Autodesk Fusion 360 part; units mm, degrees
(part 2 of 5)
sketch "Rear engraving master - manufacturing sketch" plane through (0, 0, -4.775) normal (0, 0, 1) x (1, 0, 0) in component "02 Clear acrylic"
  line L0 (17.075, 29.8895) -> (17.0879, 30.5633)
  line L1 (17.0879, 30.5633) -> (17.1264, 31.2094)
  line L2 (17.1264, 31.2094) -> (17.1907, 31.8279)
  line L3 (17.1907, 31.8279) -> (17.2807, 32.4188)
  line L4 (17.2807, 32.4188) -> (17.3964, 32.9821)
  line L5 (17.3964, 32.9821) -> (17.5378, 33.5177)
  line L6 (17.5378, 33.5177) -> (17.7049, 34.0257)
  line L7 (17.7049, 34.0257) -> (17.8977, 34.5061)
  line L8 (17.8977, 34.5061) -> (18.2326, 35.1761)
  line L9 (18.2326, 35.1761) -> (18.6236, 35.8107)
  line L10 (18.6236, 35.8107) -> (19.0706, 36.41)
  line L11 (19.0706, 36.41) -> (19.5737, 36.9741)
  line L12 (19.5737, 36.9741) -> (20.1174, 37.4852)
  line L13 (20.1174, 37.4852) -> (20.6864, 37.9256)
  line L14 (20.6864, 37.9256) -> (21.2807, 38.2955)
  line L15 (21.2807, 38.2955) -> (21.9004, 38.5948)
  line L16 (21.9004, 38.5948) -> (22.329, 38.7617)
  line L17 (22.329, 38.7617) -> (22.7737, 38.9064)
  line L18 (22.7737, 38.9064) -> (23.2345, 39.0288)
  line L19 (23.2345, 39.0288) -> (23.7115, 39.1289)
  line L20 (23.7115, 39.1289) -> (24.2045, 39.2068)
  line L21 (24.2045, 39.2068) -> (24.7137, 39.2624)
  line L22 (24.7137, 39.2624) -> (25.239, 39.2958)
  line L23 (25.239, 39.2958) -> (25.7804, 39.307)
  line L24 (25.7804, 39.307) -> (26.2714, 39.2973)
  line L25 (26.2714, 39.2973) -> (26.7501, 39.2684)
  line L26 (26.7501, 39.2684) -> (27.2163, 39.2202)
  line L27 (27.2163, 39.2202) -> (27.6701, 39.1527)
  line L28 (27.6701, 39.1527) -> (28.1114, 39.0659)
  line L29 (28.1114, 39.0659) -> (28.5404, 38.9599)
  line L30 (28.5404, 38.9599) -> (28.9569, 38.8346)
  line L31 (28.9569, 38.8346) -> (29.361, 38.69)
  line L32 (29.361, 38.69) -> (29.7527, 38.5261)
  line L33 (29.7527, 38.5261) -> (30.132, 38.3429)
  line L34 (30.132, 38.3429) -> (30.4988, 38.1405)
  line L35 (30.4988, 38.1405) -> (30.8532, 37.9187)
  line L36 (30.8532, 37.9187) -> (31.1952, 37.6777)
  line L37 (31.1952, 37.6777) -> (31.5248, 37.4174)
  line L38 (31.5248, 37.4174) -> (31.8419, 37.1379)
  line L39 (31.8419, 37.1379) -> (32.1467, 36.839)
  line L40 (32.1467, 36.839) -> (32.4358, 36.523)
  line L41 (32.4358, 36.523) -> (32.7064, 36.1919)
  line L42 (32.7064, 36.1919) -> (32.9582, 35.8458)
  line L43 (32.9582, 35.8458) -> (33.1915, 35.4846)
  line L44 (33.1915, 35.4846) -> (33.406, 35.1083)
  line L45 (33.406, 35.1083) -> (33.6019, 34.717)
  line L46 (33.6019, 34.717) -> (33.7792, 34.3106)
  line L47 (33.7792, 34.3106) -> (33.9378, 33.8892)
  line L48 (33.9378, 33.8892) -> (34.0777, 33.4526)
  line L49 (34.0777, 33.4526) -> (34.199, 33.0011)
  line L50 (34.199, 33.0011) -> (34.3016, 32.5345)
  line L51 (34.3016, 32.5345) -> (34.3855, 32.0528)
  line L52 (34.3855, 32.0528) -> (34.4508, 31.556)
  line L53 (34.4508, 31.556) -> (34.4975, 31.0442)
  line L54 (34.4975, 31.0442) -> (34.5255, 30.5174)
  line L55 (34.5255, 30.5174) -> (34.5348, 29.9754)
  line L56 (34.5348, 29.9754) -> (34.5255, 29.438)
  line L57 (34.5255, 29.438) -> (34.4978, 28.9154)
  line L58 (34.4978, 28.9154) -> (34.4515, 28.4076)
  line L59 (34.4515, 28.4076) -> (34.3867, 27.9146)
  line L60 (34.3867, 27.9146) -> (34.3034, 27.4364)
  line L61 (34.3034, 27.4364) -> (34.2015, 26.9731)
  line L62 (34.2015, 26.9731) -> (34.0812, 26.5246)
  line L63 (34.0812, 26.5246) -> (33.9424, 26.0909)
  line L64 (33.9424, 26.0909) -> (33.785, 25.672)
  line L65 (33.785, 25.672) -> (33.6091, 25.268)
  line L66 (33.6091, 25.268) -> (33.4147, 24.8787)
  line L67 (33.4147, 24.8787) -> (33.2018, 24.5043)
  line L68 (33.2018, 24.5043) -> (32.9704, 24.1447)
  line L69 (32.9704, 24.1447) -> (32.7205, 23.7999)
  line L70 (32.7205, 23.7999) -> (32.452, 23.47)
  line L71 (32.452, 23.47) -> (32.1651, 23.1548)
  line L72 (32.1651, 23.1548) -> (31.8626, 22.8567)
  line L73 (31.8626, 22.8567) -> (31.5477, 22.5779)
  line L74 (31.5477, 22.5779) -> (31.2203, 22.3182)
  line L75 (31.2203, 22.3182) -> (30.8805, 22.0778)
  line L76 (30.8805, 22.0778) -> (30.5281, 21.8566)
  line L77 (30.5281, 21.8566) -> (30.1633, 21.6547)
  line L78 (30.1633, 21.6547) -> (29.7861, 21.472)
  line L79 (29.7861, 21.472) -> (29.3963, 21.3085)
  line L80 (29.3963, 21.3085) -> (28.9941, 21.1642)
  line L81 (28.9941, 21.1642) -> (28.5794, 21.0392)
  line L82 (28.5794, 21.0392) -> (28.1523, 20.9335)
  line L83 (28.1523, 20.9335) -> (27.7127, 20.8469)
  line L84 (27.7127, 20.8469) -> (27.2606, 20.7796)
  line L85 (27.2606, 20.7796) -> (26.796, 20.7315)
  line L86 (26.796, 20.7315) -> (26.319, 20.7027)
  line L87 (26.319, 20.7027) -> (25.8295, 20.693)
  line L88 (25.8295, 20.693) -> (25.334, 20.7026)
  line L89 (25.334, 20.7026) -> (24.8514, 20.7313)
  line L90 (24.8514, 20.7313) -> (24.3817, 20.7792)
  line L91 (24.3817, 20.7792) -> (23.9248, 20.8461)
  line L92 (23.9248, 20.8461) -> (23.4808, 20.9323)
  line L93 (23.4808, 20.9323) -> (23.0496, 21.0375)
  line L94 (23.0496, 21.0375) -> (22.6313, 21.1619)
  line L95 (22.6313, 21.1619) -> (22.2258, 21.3054)
  line L96 (22.2258, 21.3054) -> (21.8332, 21.4681)
  line L97 (21.8332, 21.4681) -> (21.4534, 21.6499)
  line L98 (21.4534, 21.6499) -> (21.0865, 21.8508)
  line L99 (21.0865, 21.8508) -> (20.7324, 22.0709)
  line L100 (20.7324, 22.0709) -> (20.3912, 22.3101)
  line L101 (20.3912, 22.3101) -> (20.0629, 22.5685)
  line L102 (20.0629, 22.5685) -> (19.7474, 22.8459)
  line L103 (19.7474, 22.8459) -> (19.4447, 23.1426)
  line L104 (19.4447, 23.1426) -> (19.1578, 23.456)
  line L105 (19.1578, 23.456) -> (18.8893, 23.7838)
  line L106 (18.8893, 23.7838) -> (18.6394, 24.1261)
  line L107 (18.6394, 24.1261) -> (18.408, 24.4828)
  line L108 (18.408, 24.4828) -> (18.1951, 24.854)
  line L109 (18.1951, 24.854) -> (18.0007, 25.2396)
  line L110 (18.0007, 25.2396) -> (17.8248, 25.6396)
  line L111 (17.8248, 25.6396) -> (17.6675, 26.0541)
  line L112 (17.6675, 26.0541) -> (17.5286, 26.483)
  line L113 (17.5286, 26.483) -> (17.4083, 26.9263)
  line L114 (17.4083, 26.9263) -> (17.3065, 27.3841)
  line L115 (17.3065, 27.3841) -> (17.2231, 27.8563)
  line L116 (17.2231, 27.8563) -> (17.1583, 28.3429)
  line L117 (17.1583, 28.3429) -> (17.1121, 28.844)
  line L118 (17.1121, 28.844) -> (17.0843, 29.3595)
  line L119 (17.0843, 29.3595) -> (17.075, 29.8895)
  line L120 (20.8199, 30.0123) -> (20.842, 29.2711)
  line L121 (20.842, 29.2711) -> (20.9082, 28.5761)
  line L122 (20.9082, 28.5761) -> (21.0185, 27.9274)
  line L123 (21.0185, 27.9274) -> (21.1729, 27.3249)
  line L124 (21.1729, 27.3249) -> (21.3715, 26.7686)
  line L125 (21.3715, 26.7686) -> (21.6142, 26.2586)
  line L126 (21.6142, 26.2586) -> (21.901, 25.7948)
  line L127 (21.901, 25.7948) -> (22.2319, 25.3772)
  line L128 (22.2319, 25.3772) -> (22.5968, 25.0074)
  line L129 (22.5968, 25.0074) -> (22.9855, 24.6869)
  line L130 (22.9855, 24.6869) -> (23.398, 24.4158)
  line L131 (23.398, 24.4158) -> (23.8342, 24.1939)
  line L132 (23.8342, 24.1939) -> (24.2943, 24.0213)
  line L133 (24.2943, 24.0213) -> (24.7781, 23.8981)
  line L134 (24.7781, 23.8981) -> (25.2858, 23.8241)
  line L135 (25.2858, 23.8241) -> (25.8172, 23.7995)
  line L136 (25.8172, 23.7995) -> (26.3483, 23.8239)
  line L137 (26.3483, 23.8239) -> (26.8551, 23.8973)
  line L138 (26.8551, 23.8973) -> (27.3375, 24.0196)
  line L139 (27.3375, 24.0196) -> (27.7955, 24.1908)
  line L140 (27.7955, 24.1908) -> (28.2292, 24.411)
  line L141 (28.2292, 24.411) -> (28.6385, 24.68)
  line L142 (28.6385, 24.68) -> (29.0235, 24.998)
  line L143 (29.0235, 24.998) -> (29.384, 25.3649)
  line L144 (29.384, 25.3649) -> (29.7107, 25.7808)
  line L145 (29.7107, 25.7808) -> (29.9937, 26.2455)
  line L146 (29.9937, 26.2455) -> (30.2333, 26.7592)
  line L147 (30.2333, 26.7592) -> (30.4292, 27.3218)
  line L148 (30.4292, 27.3218) -> (30.5817, 27.9333)
  line L149 (30.5817, 27.9333) -> (30.6905, 28.5937)
  line L150 (30.6905, 28.5937) -> (30.7558, 29.3031)
  line L151 (30.7558, 29.3031) -> (30.7776, 30.0614)
  line L152 (30.7776, 30.0614) -> (30.7564, 30.8104)
  line L153 (30.7564, 30.8104) -> (30.6928, 31.5102)
  line L154 (30.6928, 31.5102) -> (30.5868, 32.161)
  line L155 (30.5868, 32.161) -> (30.4384, 32.7626)
  line L156 (30.4384, 32.7626) -> (30.2476, 33.3151)
  line L157 (30.2476, 33.3151) -> (30.0145, 33.8186)
  line L158 (30.0145, 33.8186) -> (29.7389, 34.2728)
  line L159 (29.7389, 34.2728) -> (29.4209, 34.678)
  line L160 (29.4209, 34.678) -> (29.0678, 35.0349)
  line L161 (29.0678, 35.0349) -> (28.6869, 35.3441)
  line L162 (28.6869, 35.3441) -> (28.2781, 35.6058)
  line L163 (28.2781, 35.6058) -> (27.8416, 35.8199)
  line L164 (27.8416, 35.8199) -> (27.3772, 35.9864)
  line L165 (27.3772, 35.9864) -> (26.885, 36.1054)
  line L166 (26.885, 36.1054) -> (26.365, 36.1768)
  line L167 (26.365, 36.1768) -> (25.8172, 36.2005)
  line L168 (25.8172, 36.2005) -> (25.2691, 36.1765)
  line L169 (25.2691, 36.1765) -> (24.7482, 36.1042)
  line L170 (24.7482, 36.1042) -> (24.2546, 35.9839)
  line L171 (24.2546, 35.9839) -> (23.7882, 35.8153)
  line L172 (23.7882, 35.8153) -> (23.3491, 35.5986)
  line L173 (23.3491, 35.5986) -> (22.9372, 35.3338)
  line L174 (22.9372, 35.3338) -> (22.5525, 35.0208)
  line L175 (22.5525, 35.0208) -> (22.1951, 34.6596)
  line L176 (22.1951, 34.6596) -> (21.8728, 34.2499)
  line L177 (21.8728, 34.2499) -> (21.5935, 33.7913)
  line L178 (21.5935, 33.7913) -> (21.3571, 33.2838)
  line L179 (21.3571, 33.2838) -> (21.1637, 32.7273)
  line L180 (21.1637, 32.7273) -> (21.0133, 32.1219)
  line L181 (21.0133, 32.1219) -> (20.9059, 31.4676)
  line L182 (20.9059, 31.4676) -> (20.8414, 30.7644)
  line L183 (20.8414, 30.7644) -> (20.8199, 30.0123)
  line L184 (37.4079, 21) -> (37.4079, 39)
  line L185 (37.4079, 39) -> (40.9441, 39)
  line L186 (40.9441, 39) -> (48.311, 26.9795)
  line L187 (48.311, 26.9795) -> (48.311, 39)
  line L188 (48.311, 39) -> (51.6876, 39)
  line L189 (51.6876, 39) -> (51.6876, 21)
  line L190 (51.6876, 21) -> (48.0409, 21)
  line L191 (48.0409, 21) -> (40.7844, 32.7381)
  line L192 (40.7844, 32.7381) -> (40.7844, 21)
  line L193 (40.7844, 21) -> (37.4079, 21)
  line L194 (77.8158, 21) -> (73.8622, 21)
  line L195 (73.8622, 21) -> (72.2906, 25.0887)
  line L196 (72.2906, 25.0887) -> (65.0955, 25.0887)
  line L197 (65.0955, 25.0887) -> (63.6098, 21)
  line L198 (63.6098, 21) -> (59.7544, 21)
  line L199 (59.7544, 21) -> (66.7653, 39)
  line L200 (66.7653, 39) -> (70.6085, 39)
  line L201 (70.6085, 39) -> (77.8158, 21)
  line L202 (71.1241, 28.1214) -> (68.6439, 34.8008)
  line L203 (68.6439, 34.8008) -> (66.2128, 28.1214)
  line L204 (66.2128, 28.1214) -> (71.1241, 28.1214)
  line L205 (79.633, 21) -> (79.633, 39)
  line L206 (79.633, 39) -> (83.2674, 39)
  line L207 (83.2674, 39) -> (83.2674, 21)
  line L208 (83.2674, 21) -> (79.633, 21)
  line L209 (86.7422, 21) -> (86.7422, 39)
  line L210 (86.7422, 39) -> (94.3915, 39)
  line L211 (94.3915, 39) -> (95.0882, 38.9924)
  line L212 (95.0882, 38.9924) -> (95.7356, 38.9697)
  line L213 (95.7356, 38.9697) -> (96.3337, 38.9318)
  line L214 (96.3337, 38.9318) -> (96.8825, 38.8787)
  line L215 (96.8825, 38.8787) -> (97.382, 38.8105)
  line L216 (97.382, 38.8105) -> (97.8321, 38.7272)
  line L217 (97.8321, 38.7272) -> (98.233, 38.6287)
  line L218 (98.233, 38.6287) -> (98.5846, 38.515)
  line L219 (98.5846, 38.515) -> (98.9033, 38.382)
  line L220 (98.9033, 38.382) -> (99.2058, 38.2253)
  line L221 (99.2058, 38.2253) -> (99.4919, 38.0451)
  line L222 (99.4919, 38.0451) -> (99.7618, 37.8412)
  line L223 (99.7618, 37.8412) -> (100.0153, 37.6138)
  line L224 (100.0153, 37.6138) -> (100.2525, 37.3628)
  line L225 (100.2525, 37.3628) -> (100.4734, 37.0881)
  line L226 (100.4734, 37.0881) -> (100.678, 36.7899)
  line L227 (100.678, 36.7899) -> (100.8622, 36.4743)
  line L228 (100.8622, 36.4743) -> (101.0218, 36.1476)
  line L229 (101.0218, 36.1476) -> (101.1569, 35.8097)
  line L230 (101.1569, 35.8097) -> (101.2674, 35.4608)
  line L231 (101.2674, 35.4608) -> (101.3533, 35.1007)
  line L232 (101.3533, 35.1007) -> (101.4147, 34.7294)
  line L233 (101.4147, 34.7294) -> (101.4516, 34.3471)
  line L234 (101.4516, 34.3471) -> (101.4638, 33.9536)
  line L235 (101.4638, 33.9536) -> (101.4452, 33.4582)
  line L236 (101.4452, 33.4582) -> (101.3894, 32.9848)
  line L237 (101.3894, 32.9848) -> (101.2964, 32.5335)
  line L238 (101.2964, 32.5335) -> (101.1661, 32.1042)
  line L239 (101.1661, 32.1042) -> (100.9986, 31.697)
  line L240 (100.9986, 31.697) -> (100.7939, 31.3119)
  line L241 (100.7939, 31.3119) -> (100.552, 30.9488)
  line L242 (100.552, 30.9488) -> (100.2728, 30.6078)
  line L243 (100.2728, 30.6078) -> (99.9567, 30.293)
  line L244 (99.9567, 30.293) -> (99.6037, 30.0088)
  line L245 (99.6037, 30.0088) -> (99.2138, 29.7551)
  line L246 (99.2138, 29.7551) -> (98.7872, 29.5319)
  line L247 (98.7872, 29.5319) -> (98.3237, 29.3392)
  line L248 (98.3237, 29.3392) -> (97.8233, 29.177)
  line L249 (97.8233, 29.177) -> (97.2861, 29.0453)
  line L250 (97.2861, 29.0453) -> (96.7121, 28.9441)
  line L251 (96.7121, 28.9441) -> (97.2758, 28.5918)
  line L252 (97.2758, 28.5918) -> (97.788, 28.2227)
  line L253 (97.788, 28.2227) -> (98.2488, 27.8367)
  line L254 (98.2488, 27.8367) -> (98.6582, 27.4338)
  line L255 (98.6582, 27.4338) -> (98.8584, 27.2082)
  line L256 (98.8584, 27.2082) -> (99.0753, 26.9427)
  line L257 (99.0753, 26.9427) -> (99.3089, 26.6373)
  line L258 (99.3089, 26.6373) -> (99.5592, 26.2919)
  line L259 (99.5592, 26.2919) -> (99.8261, 25.9067)
  line L260 (99.8261, 25.9067) -> (100.1098, 25.4816)
  line L261 (100.1098, 25.4816) -> (100.4101, 25.0165)
  line L262 (100.4101, 25.0165) -> (100.7271, 24.5116)
  line L263 (100.7271, 24.5116) -> (102.925, 21)
  line L264 (102.925, 21) -> (98.5784, 21)
  line L265 (98.5784, 21) -> (95.9509, 24.9168)
  line L266 (95.9509, 24.9168) -> (95.6148, 25.4174)
  line L267 (95.6148, 25.4174) -> (95.3063, 25.8695)
  line L268 (95.3063, 25.8695) -> (95.0254, 26.2731)
  line L269 (95.0254, 26.2731) -> (94.7722, 26.6281)
  line L270 (94.7722, 26.6281) -> (94.5465, 26.9345)
  line L271 (94.5465, 26.9345) -> (94.3486, 27.1925)
  line L272 (94.3486, 27.1925) -> (94.1782, 27.4019)
  line L273 (94.1782, 27.4019) -> (94.0355, 27.5628)
  line L274 (94.0355, 27.5628) -> (93.7738, 27.8145)
  line L275 (93.7738, 27.8145) -> (93.5044, 28.0232)
  line L276 (93.5044, 28.0232) -> (93.2274, 28.1889)
  line L277 (93.2274, 28.1889) -> (92.9427, 28.3117)
  line L278 (92.9427, 28.3117) -> (92.7879, 28.3592)
  line L279 (92.7879, 28.3592) -> (92.612, 28.4004)
  line L280 (92.612, 28.4004) -> (92.4149, 28.4352)
  line L281 (92.4149, 28.4352) -> (92.1968, 28.4637)
  line L282 (92.1968, 28.4637) -> (91.9576, 28.4858)
  line L283 (91.9576, 28.4858) -> (91.6972, 28.5017)
  line L284 (91.6972, 28.5017) -> (91.4158, 28.5112)
  line L285 (91.4158, 28.5112) -> (91.1132, 28.5143)
  line L286 (91.1132, 28.5143) -> (90.3765, 28.5143)
  line L287 (90.3765, 28.5143) -> (90.3765, 21)
  line L288 (90.3765, 21) -> (86.7422, 21)
  line L289 (90.3765, 31.3874) -> (93.0655, 31.3874)
  line L290 (93.0655, 31.3874) -> (93.6886, 31.3909)
  line L291 (93.6886, 31.3909) -> (94.2503, 31.4013)
  line L292 (94.2503, 31.4013) -> (94.7507, 31.4185)
  line L293 (94.7507, 31.4185) -> (95.1896, 31.4427)
  line L294 (95.1896, 31.4427) -> (95.5672, 31.4738)
  line L295 (95.5672, 31.4738) -> (95.8834, 31.5118)
  line L296 (95.8834, 31.5118) -> (96.1381, 31.5567)
  line L297 (96.1381, 31.5567) -> (96.3315, 31.6085)
  line L298 (96.3315, 31.6085) -> (96.6392, 31.7389)
  line L299 (96.6392, 31.7389) -> (96.9117, 31.9093)
  line L300 (96.9117, 31.9093) -> (97.1488, 32.1195)
  line L301 (97.1488, 32.1195) -> (97.3506, 32.3697)
  line L302 (97.3506, 32.3697) -> (97.5118, 32.6567)
  line L303 (97.5118, 32.6567) -> (97.6269, 32.9775)
  line L304 (97.6269, 32.9775) -> (97.6959, 33.332)
  line L305 (97.6959, 33.332) -> (97.719, 33.7203)
  line L306 (97.719, 33.7203) -> (97.6886, 34.1528)
  line L307 (97.6886, 34.1528) -> (97.5977, 34.5414)
  line L308 (97.5977, 34.5414) -> (97.4461, 34.8864)
  line L309 (97.4461, 34.8864) -> (97.234, 35.1876)
  line L310 (97.234, 35.1876) -> (96.9665, 35.4412)
  line L311 (96.9665, 35.4412) -> (96.6492, 35.6434)
  line L312 (96.6492, 35.6434) -> (96.282, 35.7942)
  line L313 (96.282, 35.7942) -> (95.8649, 35.8936)
  line L314 (95.8649, 35.8936) -> (95.7268, 35.908)
  line L315 (95.7268, 35.908) -> (95.5334, 35.9204)
  line L316 (95.5334, 35.9204) -> (95.2848, 35.931)
  line L317 (95.2848, 35.931) -> (94.9809, 35.9396)
  line L318 (94.9809, 35.9396) -> (94.6218, 35.9463)
  line L319 (94.6218, 35.9463) -> (94.2074, 35.9511)
  line L320 (94.2074, 35.9511) -> (93.7377, 35.954)
  line L321 (93.7377, 35.954) -> (93.2128, 35.955)
  line L322 (93.2128, 35.955) -> (90.3765, 35.955)
  line L323 (90.3765, 35.955) -> (90.3765, 31.3874)
ref_plane "WorkPlane1" through (0, 0, -5.675) normal (0, 0, 1) x (1, 0, 0) in component "03 Registered graphic backing"
sketch "Keyed graphic outline" plane through (0, 0, -5.675) normal (0, 0, 1) x (1, 0, 0) in component "03 Registered graphic backing"
  line L0 (8, 11) -> (112, 11)
  line L1 (112, 11) -> (112, 49)
  line L2 (112, 49) -> (11, 49)
  line L3 (11, 49) -> (8, 46)
  line L4 (8, 46) -> (8, 11)
extrude "Black substrate" add sketch "Keyed graphic outline" against normal blind 1.6 separate body makes body 35 in component "03 Registered graphic backing"
ref_plane "WorkPlane2" through (0, 0, -5.675) normal (0, 0, 1) x (1, 0, 0) in component "03 Registered graphic backing"
sketch "Letter outer 0" plane through (0, 0, -5.675) normal (0, 0, 1) x (1, 0, 0) in component "03 Registered graphic backing"
  line L0 (17.075, 29.8895) -> (17.0879, 30.5633)
  line L1 (17.0879, 30.5633) -> (17.1264, 31.2094)
  line L2 (17.1264, 31.2094) -> (17.1907, 31.8279)
  line L3 (17.1907, 31.8279) -> (17.2807, 32.4188)
  line L4 (17.2807, 32.4188) -> (17.3964, 32.9821)
  line L5 (17.3964, 32.9821) -> (17.5378, 33.5177)
  line L6 (17.5378, 33.5177) -> (17.7049, 34.0257)
  line L7 (17.7049, 34.0257) -> (17.8977, 34.5061)
  line L8 (17.8977, 34.5061) -> (18.2326, 35.1761)
  line L9 (18.2326, 35.1761) -> (18.6236, 35.8107)
  line L10 (18.6236, 35.8107) -> (19.0706, 36.41)
  line L11 (19.0706, 36.41) -> (19.5737, 36.9741)
  line L12 (19.5737, 36.9741) -> (20.1174, 37.4852)
  line L13 (20.1174, 37.4852) -> (20.6864, 37.9256)
  line L14 (20.6864, 37.9256) -> (21.2807, 38.2955)
  line L15 (21.2807, 38.2955) -> (21.9004, 38.5948)
  line L16 (21.9004, 38.5948) -> (22.329, 38.7617)
  line L17 (22.329, 38.7617) -> (22.7737, 38.9064)
  line L18 (22.7737, 38.9064) -> (23.2345, 39.0288)
  line L19 (23.2345, 39.0288) -> (23.7115, 39.1289)
  line L20 (23.7115, 39.1289) -> (24.2045, 39.2068)
  line L21 (24.2045, 39.2068) -> (24.7137, 39.2624)
  line L22 (24.7137, 39.2624) -> (25.239, 39.2958)
  line L23 (25.239, 39.2958) -> (25.7804, 39.307)
  line L24 (25.7804, 39.307) -> (26.2714, 39.2973)
  line L25 (26.2714, 39.2973) -> (26.7501, 39.2684)
  line L26 (26.7501, 39.2684) -> (27.2163, 39.2202)
  line L27 (27.2163, 39.2202) -> (27.6701, 39.1527)
  line L28 (27.6701, 39.1527) -> (28.1114, 39.0659)
  line L29 (28.1114, 39.0659) -> (28.5404, 38.9599)
  line L30 (28.5404, 38.9599) -> (28.9569, 38.8346)
  line L31 (28.9569, 38.8346) -> (29.361, 38.69)
  line L32 (29.361, 38.69) -> (29.7527, 38.5261)
  line L33 (29.7527, 38.5261) -> (30.132, 38.3429)
  line L34 (30.132, 38.3429) -> (30.4988, 38.1405)
  line L35 (30.4988, 38.1405) -> (30.8532, 37.9187)
  line L36 (30.8532, 37.9187) -> (31.1952, 37.6777)
  line L37 (31.1952, 37.6777) -> (31.5248, 37.4174)
  line L38 (31.5248, 37.4174) -> (31.8419, 37.1379)
  line L39 (31.8419, 37.1379) -> (32.1467, 36.839)
  line L40 (32.1467, 36.839) -> (32.4358, 36.523)
  line L41 (32.4358, 36.523) -> (32.7064, 36.1919)
  line L42 (32.7064, 36.1919) -> (32.9582, 35.8458)
  line L43 (32.9582, 35.8458) -> (33.1915, 35.4846)
  line L44 (33.1915, 35.4846) -> (33.406, 35.1083)
  line L45 (33.406, 35.1083) -> (33.6019, 34.717)
  line L46 (33.6019, 34.717) -> (33.7792, 34.3106)
  line L47 (33.7792, 34.3106) -> (33.9378, 33.8892)
  line L48 (33.9378, 33.8892) -> (34.0777, 33.4526)
  line L49 (34.0777, 33.4526) -> (34.199, 33.0011)
  line L50 (34.199, 33.0011) -> (34.3016, 32.5345)
  line L51 (34.3016, 32.5345) -> (34.3855, 32.0528)
  line L52 (34.3855, 32.0528) -> (34.4508, 31.556)
  line L53 (34.4508, 31.556) -> (34.4975, 31.0442)
  line L54 (34.4975, 31.0442) -> (34.5255, 30.5174)
  line L55 (34.5255, 30.5174) -> (34.5348, 29.9754)
  line L56 (34.5348, 29.9754) -> (34.5255, 29.438)
  line L57 (34.5255, 29.438) -> (34.4978, 28.9154)
  line L58 (34.4978, 28.9154) -> (34.4515, 28.4076)
  line L59 (34.4515, 28.4076) -> (34.3867, 27.9146)
  line L60 (34.3867, 27.9146) -> (34.3034, 27.4364)
  line L61 (34.3034, 27.4364) -> (34.2015, 26.9731)
  line L62 (34.2015, 26.9731) -> (34.0812, 26.5246)
  line L63 (34.0812, 26.5246) -> (33.9424, 26.0909)
  line L64 (33.9424, 26.0909) -> (33.785, 25.672)
  line L65 (33.785, 25.672) -> (33.6091, 25.268)
  line L66 (33.6091, 25.268) -> (33.4147, 24.8787)
  line L67 (33.4147, 24.8787) -> (33.2018, 24.5043)
  line L68 (33.2018, 24.5043) -> (32.9704, 24.1447)
  line L69 (32.9704, 24.1447) -> (32.7205, 23.7999)
  line L70 (32.7205, 23.7999) -> (32.452, 23.47)
  line L71 (32.452, 23.47) -> (32.1651, 23.1548)
  line L72 (32.1651, 23.1548) -> (31.8626, 22.8567)
  line L73 (31.8626, 22.8567) -> (31.5477, 22.5779)
  line L74 (31.5477, 22.5779) -> (31.2203, 22.3182)
  line L75 (31.2203, 22.3182) -> (30.8805, 22.0778)
  line L76 (30.8805, 22.0778) -> (30.5281, 21.8566)
  line L77 (30.5281, 21.8566) -> (30.1633, 21.6547)
  line L78 (30.1633, 21.6547) -> (29.7861, 21.472)
  line L79 (29.7861, 21.472) -> (29.3963, 21.3085)
  line L80 (29.3963, 21.3085) -> (28.9941, 21.1642)
  line L81 (28.9941, 21.1642) -> (28.5794, 21.0392)
  line L82 (28.5794, 21.0392) -> (28.1523, 20.9335)
  line L83 (28.1523, 20.9335) -> (27.7127, 20.8469)
  line L84 (27.7127, 20.8469) -> (27.2606, 20.7796)
  line L85 (27.2606, 20.7796) -> (26.796, 20.7315)
  line L86 (26.796, 20.7315) -> (26.319, 20.7027)
  line L87 (26.319, 20.7027) -> (25.8295, 20.693)
  line L88 (25.8295, 20.693) -> (25.334, 20.7026)
  line L89 (25.334, 20.7026) -> (24.8514, 20.7313)
  line L90 (24.8514, 20.7313) -> (24.3817, 20.7792)
  line L91 (24.3817, 20.7792) -> (23.9248, 20.8461)
  line L92 (23.9248, 20.8461) -> (23.4808, 20.9323)
  line L93 (23.4808, 20.9323) -> (23.0496, 21.0375)
  line L94 (23.0496, 21.0375) -> (22.6313, 21.1619)
  line L95 (22.6313, 21.1619) -> (22.2258, 21.3054)
  line L96 (22.2258, 21.3054) -> (21.8332, 21.4681)
  line L97 (21.8332, 21.4681) -> (21.4534, 21.6499)
  line L98 (21.4534, 21.6499) -> (21.0865, 21.8508)
  line L99 (21.0865, 21.8508) -> (20.7324, 22.0709)
  line L100 (20.7324, 22.0709) -> (20.3912, 22.3101)
  line L101 (20.3912, 22.3101) -> (20.0629, 22.5685)
  line L102 (20.0629, 22.5685) -> (19.7474, 22.8459)
  line L103 (19.7474, 22.8459) -> (19.4447, 23.1426)
  line L104 (19.4447, 23.1426) -> (19.1578, 23.456)
  line L105 (19.1578, 23.456) -> (18.8893, 23.7838)
  line L106 (18.8893, 23.7838) -> (18.6394, 24.1261)
  line L107 (18.6394, 24.1261) -> (18.408, 24.4828)
  line L108 (18.408, 24.4828) -> (18.1951, 24.854)
  line L109 (18.1951, 24.854) -> (18.0007, 25.2396)
  line L110 (18.0007, 25.2396) -> (17.8248, 25.6396)
  line L111 (17.8248, 25.6396) -> (17.6675, 26.0541)
  line L112 (17.6675, 26.0541) -> (17.5286, 26.483)
  line L113 (17.5286, 26.483) -> (17.4083, 26.9263)
  line L114 (17.4083, 26.9263) -> (17.3065, 27.3841)
  line L115 (17.3065, 27.3841) -> (17.2231, 27.8563)
  line L116 (17.2231, 27.8563) -> (17.1583, 28.3429)
  line L117 (17.1583, 28.3429) -> (17.1121, 28.844)
  line L118 (17.1121, 28.844) -> (17.0843, 29.3595)
  line L119 (17.0843, 29.3595) -> (17.075, 29.8895)
extrude "Raised letter 0" add sketch "Letter outer 0" along normal blind 0.4 separate body makes body 36 in component "03 Registered graphic backing"
ref_plane "WorkPlane3" through (0, 0, -5.675) normal (0, 0, 1) x (1, 0, 0) in component "03 Registered graphic backing"
sketch "Letter outer 2" plane through (0, 0, -5.675) normal (0, 0, 1) x (1, 0, 0) in component "03 Registered graphic backing"
  line L0 (37.4079, 21) -> (37.4079, 39)
  line L1 (37.4079, 39) -> (40.9441, 39)
  line L2 (40.9441, 39) -> (48.311, 26.9795)
  line L3 (48.311, 26.9795) -> (48.311, 39)
  line L4 (48.311, 39) -> (51.6876, 39)
  line L5 (51.6876, 39) -> (51.6876, 21)
  line L6 (51.6876, 21) -> (48.0409, 21)
  line L7 (48.0409, 21) -> (40.7844, 32.7381)
  line L8 (40.7844, 32.7381) -> (40.7844, 21)
  line L9 (40.7844, 21) -> (37.4079, 21)
extrude "Raised letter 2" add sketch "Letter outer 2" along normal blind 0.4 separate body makes body 37 in component "03 Registered graphic backing"
ref_plane "WorkPlane4" through (0, 0, -5.675) normal (0, 0, 1) x (1, 0, 0) in component "03 Registered graphic backing"
sketch "Letter outer 3" plane through (0, 0, -5.675) normal (0, 0, 1) x (1, 0, 0) in component "03 Registered graphic backing"
  line L0 (77.8158, 21) -> (73.8622, 21)
  line L1 (73.8622, 21) -> (72.2906, 25.0887)
  line L2 (72.2906, 25.0887) -> (65.0955, 25.0887)
  line L3 (65.0955, 25.0887) -> (63.6098, 21)
  line L4 (63.6098, 21) -> (59.7544, 21)
  line L5 (59.7544, 21) -> (66.7653, 39)
  line L6 (66.7653, 39) -> (70.6085, 39)
  line L7 (70.6085, 39) -> (77.8158, 21)
extrude "Raised letter 3" add sketch "Letter outer 3" along normal blind 0.4 separate body makes body 38 in component "03 Registered graphic backing"
ref_plane "WorkPlane5" through (0, 0, -5.675) normal (0, 0, 1) x (1, 0, 0) in component "03 Registered graphic backing"
sketch "Letter outer 5" plane through (0, 0, -5.675) normal (0, 0, 1) x (1, 0, 0) in component "03 Registered graphic backing"
  line L0 (79.633, 21) -> (79.633, 39)
  line L1 (79.633, 39) -> (83.2674, 39)
  line L2 (83.2674, 39) -> (83.2674, 21)
  line L3 (83.2674, 21) -> (79.633, 21)
extrude "Raised letter 5" add sketch "Letter outer 5" along normal blind 0.4 separate body makes body 39 in component "03 Registered graphic backing"
ref_plane "WorkPlane6" through (0, 0, -5.675) normal (0, 0, 1) x (1, 0, 0) in component "03 Registered graphic backing"
sketch "Letter outer 6" plane through (0, 0, -5.675) normal (0, 0, 1) x (1, 0, 0) in component "03 Registered graphic backing"
  line L0 (86.7422, 21) -> (86.7422, 39)
  line L1 (86.7422, 39) -> (94.3915, 39)
  line L2 (94.3915, 39) -> (95.0882, 38.9924)
  line L3 (95.0882, 38.9924) -> (95.7356, 38.9697)
  line L4 (95.7356, 38.9697) -> (96.3337, 38.9318)
  line L5 (96.3337, 38.9318) -> (96.8825, 38.8787)
  line L6 (96.8825, 38.8787) -> (97.382, 38.8105)
  line L7 (97.382, 38.8105) -> (97.8321, 38.7272)
  line L8 (97.8321, 38.7272) -> (98.233, 38.6287)
  line L9 (98.233, 38.6287) -> (98.5846, 38.515)
  line L10 (98.5846, 38.515) -> (98.9033, 38.382)
  line L11 (98.9033, 38.382) -> (99.2058, 38.2253)
  line L12 (99.2058, 38.2253) -> (99.4919, 38.0451)
  line L13 (99.4919, 38.0451) -> (99.7618, 37.8412)
  line L14 (99.7618, 37.8412) -> (100.0153, 37.6138)
  line L15 (100.0153, 37.6138) -> (100.2525, 37.3628)
  line L16 (100.2525, 37.3628) -> (100.4734, 37.0881)
  line L17 (100.4734, 37.0881) -> (100.678, 36.7899)
  line L18 (100.678, 36.7899) -> (100.8622, 36.4743)
  line L19 (100.8622, 36.4743) -> (101.0218, 36.1476)
  line L20 (101.0218, 36.1476) -> (101.1569, 35.8097)
  line L21 (101.1569, 35.8097) -> (101.2674, 35.4608)
  line L22 (101.2674, 35.4608) -> (101.3533, 35.1007)
  line L23 (101.3533, 35.1007) -> (101.4147, 34.7294)
  line L24 (101.4147, 34.7294) -> (101.4516, 34.3471)
  line L25 (101.4516, 34.3471) -> (101.4638, 33.9536)
  line L26 (101.4638, 33.9536) -> (101.4452, 33.4582)
  line L27 (101.4452, 33.4582) -> (101.3894, 32.9848)
  line L28 (101.3894, 32.9848) -> (101.2964, 32.5335)
  line L29 (101.2964, 32.5335) -> (101.1661, 32.1042)
  line L30 (101.1661, 32.1042) -> (100.9986, 31.697)
  line L31 (100.9986, 31.697) -> (100.7939, 31.3119)
  line L32 (100.7939, 31.3119) -> (100.552, 30.9488)
  line L33 (100.552, 30.9488) -> (100.2728, 30.6078)
  line L34 (100.2728, 30.6078) -> (99.9567, 30.293)
  line L35 (99.9567, 30.293) -> (99.6037, 30.0088)
  line L36 (99.6037, 30.0088) -> (99.2138, 29.7551)
  line L37 (99.2138, 29.7551) -> (98.7872, 29.5319)
  line L38 (98.7872, 29.5319) -> (98.3237, 29.3392)
  line L39 (98.3237, 29.3392) -> (97.8233, 29.177)
  line L40 (97.8233, 29.177) -> (97.2861, 29.0453)
  line L41 (97.2861, 29.0453) -> (96.7121, 28.9441)
  line L42 (96.7121, 28.9441) -> (97.2758, 28.5918)
  line L43 (97.2758, 28.5918) -> (97.788, 28.2227)
  line L44 (97.788, 28.2227) -> (98.2488, 27.8367)
  line L45 (98.2488, 27.8367) -> (98.6582, 27.4338)
  line L46 (98.6582, 27.4338) -> (98.8584, 27.2082)
  line L47 (98.8584, 27.2082) -> (99.0753, 26.9427)
  line L48 (99.0753, 26.9427) -> (99.3089, 26.6373)
  line L49 (99.3089, 26.6373) -> (99.5592, 26.2919)
  line L50 (99.5592, 26.2919) -> (99.8261, 25.9067)
  line L51 (99.8261, 25.9067) -> (100.1098, 25.4816)
  line L52 (100.1098, 25.4816) -> (100.4101, 25.0165)
  line L53 (100.4101, 25.0165) -> (100.7271, 24.5116)
  line L54 (100.7271, 24.5116) -> (102.925, 21)
  line L55 (102.925, 21) -> (98.5784, 21)
  line L56 (98.5784, 21) -> (95.9509, 24.9168)
  line L57 (95.9509, 24.9168) -> (95.6148, 25.4174)
  line L58 (95.6148, 25.4174) -> (95.3063, 25.8695)
  line L59 (95.3063, 25.8695) -> (95.0254, 26.2731)
  line L60 (95.0254, 26.2731) -> (94.7722, 26.6281)
  line L61 (94.7722, 26.6281) -> (94.5465, 26.9345)
  line L62 (94.5465, 26.9345) -> (94.3486, 27.1925)
  line L63 (94.3486, 27.1925) -> (94.1782, 27.4019)
  line L64 (94.1782, 27.4019) -> (94.0355, 27.5628)
  line L65 (94.0355, 27.5628) -> (93.7738, 27.8145)
  line L66 (93.7738, 27.8145) -> (93.5044, 28.0232)
  line L67 (93.5044, 28.0232) -> (93.2274, 28.1889)
  line L68 (93.2274, 28.1889) -> (92.9427, 28.3117)
  line L69 (92.9427, 28.3117) -> (92.7879, 28.3592)
  line L70 (92.7879, 28.3592) -> (92.612, 28.4004)
  line L71 (92.612, 28.4004) -> (92.4149, 28.4352)
  line L72 (92.4149, 28.4352) -> (92.1968, 28.4637)
  line L73 (92.1968, 28.4637) -> (91.9576, 28.4858)
  line L74 (91.9576, 28.4858) -> (91.6972, 28.5017)
  line L75 (91.6972, 28.5017) -> (91.4158, 28.5112)
  line L76 (91.4158, 28.5112) -> (91.1132, 28.5143)
  line L77 (91.1132, 28.5143) -> (90.3765, 28.5143)
  line L78 (90.3765, 28.5143) -> (90.3765, 21)
  line L79 (90.3765, 21) -> (86.7422, 21)
extrude "Raised letter 6" add sketch "Letter outer 6" along normal blind 0.4 separate body makes body 40 in component "03 Registered graphic backing"
combine "Union manufactured solid'" operation add target body 35 tool bodies 36 37 38 39 40 in component "03 Registered graphic backing"
ref_plane "WorkPlane7" through (0, 0, -5.275) normal (0, 0, 1) x (1, 0, 0) in component "03 Registered graphic backing"
sketch "Letter counter 1" plane through (0, 0, -5.275) normal (0, 0, 1) x (1, 0, 0) in component "03 Registered graphic backing"
  line L0 (20.8199, 30.0123) -> (20.842, 29.2711)
  line L1 (20.842, 29.2711) -> (20.9082, 28.5761)
  line L2 (20.9082, 28.5761) -> (21.0185, 27.9274)
  line L3 (21.0185, 27.9274) -> (21.1729, 27.3249)
  line L4 (21.1729, 27.3249) -> (21.3715, 26.7686)
  line L5 (21.3715, 26.7686) -> (21.6142, 26.2586)
  line L6 (21.6142, 26.2586) -> (21.901, 25.7948)
  line L7 (21.901, 25.7948) -> (22.2319, 25.3772)
  line L8 (22.2319, 25.3772) -> (22.5968, 25.0074)
  line L9 (22.5968, 25.0074) -> (22.9855, 24.6869)
  line L10 (22.9855, 24.6869) -> (23.398, 24.4158)
  line L11 (23.398, 24.4158) -> (23.8342, 24.1939)
  line L12 (23.8342, 24.1939) -> (24.2943, 24.0213)
  line L13 (24.2943, 24.0213) -> (24.7781, 23.8981)
  line L14 (24.7781, 23.8981) -> (25.2858, 23.8241)
  line L15 (25.2858, 23.8241) -> (25.8172, 23.7995)
  line L16 (25.8172, 23.7995) -> (26.3483, 23.8239)
  line L17 (26.3483, 23.8239) -> (26.8551, 23.8973)
  line L18 (26.8551, 23.8973) -> (27.3375, 24.0196)
  line L19 (27.3375, 24.0196) -> (27.7955, 24.1908)
  line L20 (27.7955, 24.1908) -> (28.2292, 24.411)
  line L21 (28.2292, 24.411) -> (28.6385, 24.68)
  line L22 (28.6385, 24.68) -> (29.0235, 24.998)
  line L23 (29.0235, 24.998) -> (29.384, 25.3649)
  line L24 (29.384, 25.3649) -> (29.7107, 25.7808)
  line L25 (29.7107, 25.7808) -> (29.9937, 26.2455)
  line L26 (29.9937, 26.2455) -> (30.2333, 26.7592)
  line L27 (30.2333, 26.7592) -> (30.4292, 27.3218)
  line L28 (30.4292, 27.3218) -> (30.5817, 27.9333)
  line L29 (30.5817, 27.9333) -> (30.6905, 28.5937)
  line L30 (30.6905, 28.5937) -> (30.7558, 29.3031)
  line L31 (30.7558, 29.3031) -> (30.7776, 30.0614)
  line L32 (30.7776, 30.0614) -> (30.7564, 30.8104)
  line L33 (30.7564, 30.8104) -> (30.6928, 31.5102)
  line L34 (30.6928, 31.5102) -> (30.5868, 32.161)
  line L35 (30.5868, 32.161) -> (30.4384, 32.7626)
  line L36 (30.4384, 32.7626) -> (30.2476, 33.3151)
  line L37 (30.2476, 33.3151) -> (30.0145, 33.8186)
  line L38 (30.0145, 33.8186) -> (29.7389, 34.2728)
  line L39 (29.7389, 34.2728) -> (29.4209, 34.678)
  line L40 (29.4209, 34.678) -> (29.0678, 35.0349)
  line L41 (29.0678, 35.0349) -> (28.6869, 35.3441)
  line L42 (28.6869, 35.3441) -> (28.2781, 35.6058)
  line L43 (28.2781, 35.6058) -> (27.8416, 35.8199)
  line L44 (27.8416, 35.8199) -> (27.3772, 35.9864)
  line L45 (27.3772, 35.9864) -> (26.885, 36.1054)
  line L46 (26.885, 36.1054) -> (26.365, 36.1768)
  line L47 (26.365, 36.1768) -> (25.8172, 36.2005)
  line L48 (25.8172, 36.2005) -> (25.2691, 36.1765)
  line L49 (25.2691, 36.1765) -> (24.7482, 36.1042)
  line L50 (24.7482, 36.1042) -> (24.2546, 35.9839)
  line L51 (24.2546, 35.9839) -> (23.7882, 35.8153)
  line L52 (23.7882, 35.8153) -> (23.3491, 35.5986)
  line L53 (23.3491, 35.5986) -> (22.9372, 35.3338)
  line L54 (22.9372, 35.3338) -> (22.5525, 35.0208)
  line L55 (22.5525, 35.0208) -> (22.1951, 34.6596)
  line L56 (22.1951, 34.6596) -> (21.8728, 34.2499)
  line L57 (21.8728, 34.2499) -> (21.5935, 33.7913)
  line L58 (21.5935, 33.7913) -> (21.3571, 33.2838)
  line L59 (21.3571, 33.2838) -> (21.1637, 32.7273)
  line L60 (21.1637, 32.7273) -> (21.0133, 32.1219)
  line L61 (21.0133, 32.1219) -> (20.9059, 31.4676)
  line L62 (20.9059, 31.4676) -> (20.8414, 30.7644)
  line L63 (20.8414, 30.7644) -> (20.8199, 30.0123)
extrude "Letter counter 1 (1)" cut sketch "Letter counter 1" against normal blind 0.4 bodies 35 in component "03 Registered graphic backing"
ref_plane "WorkPlane8" through (0, 0, -5.275) normal (0, 0, 1) x (1, 0, 0) in component "03 Registered graphic backing"
sketch "Letter counter 4" plane through (0, 0, -5.275) normal (0, 0, 1) x (1, 0, 0) in component "03 Registered graphic backing"
  line L0 (71.1241, 28.1214) -> (68.6439, 34.8008)
  line L1 (68.6439, 34.8008) -> (66.2128, 28.1214)
  line L2 (66.2128, 28.1214) -> (71.1241, 28.1214)
extrude "Letter counter 4 (1)" cut sketch "Letter counter 4" against normal blind 0.4 bodies 35 in component "03 Registered graphic backing"
ref_plane "WorkPlane9" through (0, 0, -5.275) normal (0, 0, 1) x (1, 0, 0) in component "03 Registered graphic backing"
sketch "Letter counter 7" plane through (0, 0, -5.275) normal (0, 0, 1) x (1, 0, 0) in component "03 Registered graphic backing"
  line L0 (90.3765, 31.3874) -> (93.0655, 31.3874)
  line L1 (93.0655, 31.3874) -> (93.6886, 31.3909)
  line L2 (93.6886, 31.3909) -> (94.2503, 31.4013)
  line L3 (94.2503, 31.4013) -> (94.7507, 31.4185)
  line L4 (94.7507, 31.4185) -> (95.1896, 31.4427)
  line L5 (95.1896, 31.4427) -> (95.5672, 31.4738)
  line L6 (95.5672, 31.4738) -> (95.8834, 31.5118)
  line L7 (95.8834, 31.5118) -> (96.1381, 31.5567)
  line L8 (96.1381, 31.5567) -> (96.3315, 31.6085)
  line L9 (96.3315, 31.6085) -> (96.6392, 31.7389)
  line L10 (96.6392, 31.7389) -> (96.9117, 31.9093)
  line L11 (96.9117, 31.9093) -> (97.1488, 32.1195)
  line L12 (97.1488, 32.1195) -> (97.3506, 32.3697)
  line L13 (97.3506, 32.3697) -> (97.5118, 32.6567)
  line L14 (97.5118, 32.6567) -> (97.6269, 32.9775)
  line L15 (97.6269, 32.9775) -> (97.6959, 33.332)
  line L16 (97.6959, 33.332) -> (97.719, 33.7203)
  line L17 (97.719, 33.7203) -> (97.6886, 34.1528)
  line L18 (97.6886, 34.1528) -> (97.5977, 34.5414)
  line L19 (97.5977, 34.5414) -> (97.4461, 34.8864)
  line L20 (97.4461, 34.8864) -> (97.234, 35.1876)
  line L21 (97.234, 35.1876) -> (96.9665, 35.4412)
  line L22 (96.9665, 35.4412) -> (96.6492, 35.6434)
  line L23 (96.6492, 35.6434) -> (96.282, 35.7942)
  line L24 (96.282, 35.7942) -> (95.8649, 35.8936)
  line L25 (95.8649, 35.8936) -> (95.7268, 35.908)
  line L26 (95.7268, 35.908) -> (95.5334, 35.9204)
  line L27 (95.5334, 35.9204) -> (95.2848, 35.931)
  line L28 (95.2848, 35.931) -> (94.9809, 35.9396)
  line L29 (94.9809, 35.9396) -> (94.6218, 35.9463)
  line L30 (94.6218, 35.9463) -> (94.2074, 35.9511)
  line L31 (94.2074, 35.9511) -> (93.7377, 35.954)
  line L32 (93.7377, 35.954) -> (93.2128, 35.955)
  line L33 (93.2128, 35.955) -> (90.3765, 35.955)
  line L34 (90.3765, 35.955) -> (90.3765, 31.3874)
extrude "Letter counter 7 (1)" cut sketch "Letter counter 7" against normal blind 0.4 bodies 35 in component "03 Registered graphic backing"
ref_plane "WorkPlane10" through (0, 0, -4.775) normal (0, 0, 1) x (1, 0, 0) in component "03 Registered graphic backing"
sketch "Hidden acrylic spacing pad profile" plane through (0, 0, -4.775) normal (0, 0, 1) x (1, 0, 0) in component "03 Registered graphic backing"
  line L0 (8.3, 20) -> (9.7, 20)
  line L1 (9.7, 20) -> (9.7, 26)
  line L2 (9.7, 26) -> (8.3, 26)
  line L3 (8.3, 26) -> (8.3, 20)
  dimension "d379" = 1.4
  dimension "d380" = 6
  measures "d379" horizontal distance of L0.start L0.end
  measures "d380" vertical distance of L0.end L1.end
extrude "Hidden acrylic spacing pad" add sketch "Hidden acrylic spacing pad profile" against normal blind 0.9 separate body makes body 41 in component "03 Registered graphic backing"
ref_plane "WorkPlane11" through (0, 0, -4.775) normal (0, 0, 1) x (1, 0, 0) in component "03 Registered graphic backing"
sketch "Hidden acrylic spacing pad profile (1)" plane through (0, 0, -4.775) normal (0, 0, 1) x (1, 0, 0) in component "03 Registered graphic backing"
  line L0 (8.3, 35) -> (9.7, 35)
  line L1 (9.7, 35) -> (9.7, 41)
  line L2 (9.7, 41) -> (8.3, 41)
  line L3 (8.3, 41) -> (8.3, 35)
  dimension "d385" = 1.4
  dimension "d386" = 6
  measures "d385" horizontal distance of L0.start L0.end
  measures "d386" vertical distance of L0.end L1.end
extrude "Hidden acrylic spacing pad (1)" add sketch "Hidden acrylic spacing pad profile (1)" against normal blind 0.9 separate body makes body 42 in component "03 Registered graphic backing"
ref_plane "WorkPlane12" through (0, 0, -4.775) normal (0, 0, 1) x (1, 0, 0) in component "03 Registered graphic backing"
sketch "Hidden acrylic spacing pad profile (2)" plane through (0, 0, -4.775) normal (0, 0, 1) x (1, 0, 0) in component "03 Registered graphic backing"
  line L0 (110.3, 20) -> (111.7, 20)
  line L1 (111.7, 20) -> (111.7, 26)
  line L2 (111.7, 26) -> (110.3, 26)
  line L3 (110.3, 26) -> (110.3, 20)
  dimension "d391" = 1.4
  dimension "d392" = 6
  measures "d391" horizontal distance of L0.start L0.end
  measures "d392" vertical distance of L0.end L1.end
extrude "Hidden acrylic spacing pad (2)" add sketch "Hidden acrylic spacing pad profile (2)" against normal blind 0.9 separate body makes body 43 in component "03 Registered graphic backing"
ref_plane "WorkPlane13" through (0, 0, -4.775) normal (0, 0, 1) x (1, 0, 0) in component "03 Registered graphic backing"
sketch "Hidden acrylic spacing pad profile (3)" plane through (0, 0, -4.775) normal (0, 0, 1) x (1, 0, 0) in component "03 Registered graphic backing"
  line L0 (110.3, 35) -> (111.7, 35)
  line L1 (111.7, 35) -> (111.7, 41)
  line L2 (111.7, 41) -> (110.3, 41)
  line L3 (110.3, 41) -> (110.3, 35)
  dimension "d397" = 1.4
  dimension "d398" = 6
  measures "d397" horizontal distance of L0.start L0.end
  measures "d398" vertical distance of L0.end L1.end
extrude "Hidden acrylic spacing pad (3)" add sketch "Hidden acrylic spacing pad profile (3)" against normal blind 0.9 separate body makes body 44 in component "03 Registered graphic backing"
ref_plane "WorkPlane14" through (0, 0, -4.775) normal (0, 0, 1) x (1, 0, 0) in component "03 Registered graphic backing"
sketch "Hidden acrylic spacing pad profile (4)" plane through (0, 0, -4.775) normal (0, 0, 1) x (1, 0, 0) in component "03 Registered graphic backing"
  line L0 (22, 11.3) -> (28, 11.3)
  line L1 (28, 11.3) -> (28, 12.7)
  line L2 (28, 12.7) -> (22, 12.7)
  line L3 (22, 12.7) -> (22, 11.3)
  dimension "d403" = 6
  dimension "d404" = 1.4
  measures "d403" horizontal distance of L0.start L0.end
  measures "d404" vertical distance of L0.end L1.end
extrude "Hidden acrylic spacing pad (4)" add sketch "Hidden acrylic spacing pad profile (4)" against normal blind 0.9 separate body makes body 45 in component "03 Registered graphic backing"
ref_plane "WorkPlane15" through (0, 0, -4.775) normal (0, 0, 1) x (1, 0, 0) in component "03 Registered graphic backing"
sketch "Hidden acrylic spacing pad profile (5)" plane through (0, 0, -4.775) normal (0, 0, 1) x (1, 0, 0) in component "03 Registered graphic backing"
  line L0 (38, 11.3) -> (44, 11.3)
  line L1 (44, 11.3) -> (44, 12.7)
  line L2 (44, 12.7) -> (38, 12.7)
  line L3 (38, 12.7) -> (38, 11.3)
  dimension "d409" = 6
  dimension "d410" = 1.4
  measures "d409" horizontal distance of L0.start L0.end
  measures "d410" vertical distance of L0.end L1.end
extrude "Hidden acrylic spacing pad (5)" add sketch "Hidden acrylic spacing pad profile (5)" against normal blind 0.9 separate body makes body 46 in component "03 Registered graphic backing"
ref_plane "WorkPlane16" through (0, 0, -4.775) normal (0, 0, 1) x (1, 0, 0) in component "03 Registered graphic backing"
sketch "Hidden acrylic spacing pad profile (6)" plane through (0, 0, -4.775) normal (0, 0, 1) x (1, 0, 0) in component "03 Registered graphic backing"
  line L0 (78, 11.3) -> (84, 11.3)
  line L1 (84, 11.3) -> (84, 12.7)
  line L2 (84, 12.7) -> (78, 12.7)
  line L3 (78, 12.7) -> (78, 11.3)
  dimension "d415" = 6
  dimension "d416" = 1.4
  measures "d415" horizontal distance of L0.start L0.end
  measures "d416" vertical distance of L0.end L1.end
extrude "Hidden acrylic spacing pad (6)" add sketch "Hidden acrylic spacing pad profile (6)" against normal blind 0.9 separate body makes body 47 in component "03 Registered graphic backing"
ref_plane "WorkPlane17" through (0, 0, -4.775) normal (0, 0, 1) x (1, 0, 0) in component "03 Registered graphic backing"
sketch "Hidden acrylic spacing pad profile (7)" plane through (0, 0, -4.775) normal (0, 0, 1) x (1, 0, 0) in component "03 Registered graphic backing"
  line L0 (94, 11.3) -> (100, 11.3)
  line L1 (100, 11.3) -> (100, 12.7)
  line L2 (100, 12.7) -> (94, 12.7)
  line L3 (94, 12.7) -> (94, 11.3)
  dimension "d421" = 6
  dimension "d422" = 1.4
  measures "d421" horizontal distance of L0.start L0.end
  measures "d422" vertical distance of L0.end L1.end
extrude "Hidden acrylic spacing pad (7)" add sketch "Hidden acrylic spacing pad profile (7)" against normal blind 0.9 separate body makes body 48 in component "03 Registered graphic backing"
ref_plane "WorkPlane18" through (0, 0, -4.775) normal (0, 0, 1) x (1, 0, 0) in component "03 Registered graphic backing"
sketch "Hidden acrylic spacing pad profile (8)" plane through (0, 0, -4.775) normal (0, 0, 1) x (1, 0, 0) in component "03 Registered graphic backing"
  line L0 (22, 47.3) -> (28, 47.3)
  line L1 (28, 47.3) -> (28, 48.7)
  line L2 (28, 48.7) -> (22, 48.7)
  line L3 (22, 48.7) -> (22, 47.3)
  dimension "d427" = 6
  dimension "d428" = 1.4
  measures "d427" horizontal distance of L0.start L0.end
  measures "d428" vertical distance of L0.end L1.end
extrude "Hidden acrylic spacing pad (8)" add sketch "Hidden acrylic spacing pad profile (8)" against normal blind 0.9 separate body makes body 49 in component "03 Registered graphic backing"
ref_plane "WorkPlane19" through (0, 0, -4.775) normal (0, 0, 1) x (1, 0, 0) in component "03 Registered graphic backing"
sketch "Hidden acrylic spacing pad profile (9)" plane through (0, 0, -4.775) normal (0, 0, 1) x (1, 0, 0) in component "03 Registered graphic backing"
  line L0 (38, 47.3) -> (44, 47.3)
  line L1 (44, 47.3) -> (44, 48.7)
  line L2 (44, 48.7) -> (38, 48.7)
  line L3 (38, 48.7) -> (38, 47.3)
  dimension "d433" = 6
  dimension "d434" = 1.4
  measures "d433" horizontal distance of L0.start L0.end
  measures "d434" vertical distance of L0.end L1.end
extrude "Hidden acrylic spacing pad (9)" add sketch "Hidden acrylic spacing pad profile (9)" against normal blind 0.9 separate body makes body 50 in component "03 Registered graphic backing"
ref_plane "WorkPlane20" through (0, 0, -4.775) normal (0, 0, 1) x (1, 0, 0) in component "03 Registered graphic backing"
sketch "Hidden acrylic spacing pad profile (10)" plane through (0, 0, -4.775) normal (0, 0, 1) x (1, 0, 0) in component "03 Registered graphic backing"
  line L0 (78, 47.3) -> (84, 47.3)
  line L1 (84, 47.3) -> (84, 48.7)
  line L2 (84, 48.7) -> (78, 48.7)
  line L3 (78, 48.7) -> (78, 47.3)
  dimension "d439" = 6
  dimension "d440" = 1.4
  measures "d439" horizontal distance of L0.start L0.end
  measures "d440" vertical distance of L0.end L1.end
extrude "Hidden acrylic spacing pad (10)" add sketch "Hidden acrylic spacing pad profile (10)" against normal blind 0.9 separate body makes body 51 in component "03 Registered graphic backing"
ref_plane "WorkPlane21" through (0, 0, -4.775) normal (0, 0, 1) x (1, 0, 0) in component "03 Registered graphic backing"
sketch "Hidden acrylic spacing pad profile (11)" plane through (0, 0, -4.775) normal (0, 0, 1) x (1, 0, 0) in component "03 Registered graphic backing"
  line L0 (94, 47.3) -> (100, 47.3)
  line L1 (100, 47.3) -> (100, 48.7)
  line L2 (100, 48.7) -> (94, 48.7)
  line L3 (94, 48.7) -> (94, 47.3)
  dimension "d445" = 6
  dimension "d446" = 1.4
  measures "d445" horizontal distance of L0.start L0.end
  measures "d446" vertical distance of L0.end L1.end
extrude "Hidden acrylic spacing pad (11)" add sketch "Hidden acrylic spacing pad profile (11)" against normal blind 0.9 separate body makes body 52 in component "03 Registered graphic backing"
combine "Union manufactured solid (1)'" operation add target body 35 tool bodies 41 42 43 44 45 46 47 48 49 50 51 52 in component "03 Registered graphic backing"
ref_plane "WorkPlane1" through (0, 0, -7.475) normal (0, 0, 1) x (1, 0, 0) in component "04 Optical retainer"
sketch "Perimeter retainer profile" plane through (0, 0, -7.475) normal (0, 0, 1) x (1, 0, 0) in component "04 Optical retainer"
  line L0 (8, 11) -> (112, 11)
  line L1 (112, 11) -> (112, 49)
  line L2 (112, 49) -> (8, 49)
  line L3 (8, 49) -> (8, 11)
  dimension "d451" = 104
  dimension "d452" = 38
  measures "d451" horizontal distance of L0.start L0.end
  measures "d452" vertical distance of L0.end L1.end
extrude "Perimeter retainer" add sketch "Perimeter retainer profile" against normal blind 1.6 separate body makes body 53 in component "04 Optical retainer"
ref_plane "WorkPlane2" through (0, 0, -7.455) normal (0, 0, 1) x (1, 0, 0) in component "04 Optical retainer"
sketch "Open retainer center profile" plane through (0, 0, -7.455) normal (0, 0, 1) x (1, 0, 0) in component "04 Optical retainer"
  line L0 (11, 14) -> (109, 14)
  line L1 (109, 14) -> (109, 46)
  line L2 (109, 46) -> (11, 46)
  line L3 (11, 46) -> (11, 14)
  dimension "d457" = 98
  dimension "d458" = 32
  measures "d457" horizontal distance of L0.start L0.end
  measures "d458" vertical distance of L0.end L1.end
extrude "Open retainer center" cut sketch "Open retainer center profile" against normal blind 1.64 bodies 53 in component "04 Optical retainer"
ref_plane "WorkPlane3" through (0, 0, -7.475) normal (0, 0, 1) x (1, 0, 0) in component "04 Optical retainer"
sketch "Optical screw ear profile" plane through (0, 0, -7.475) normal (0, 0, 1) x (1, 0, 0) in component "04 Optical retainer"
  line L0 (55.8, 3) -> (64.2, 3)
  line L1 (64.2, 3) -> (64.2, 13)
  line L2 (64.2, 13) -> (55.8, 13)
  line L3 (55.8, 13) -> (55.8, 3)
  dimension "d463" = 8.4
  dimension "d464" = 10
  measures "d463" horizontal distance of L0.start L0.end
  measures "d464" vertical distance of L0.end L1.end
extrude "Optical screw ear" add sketch "Optical screw ear profile" against normal blind 1.6 separate body makes body 54 in component "04 Optical retainer"
ref_plane "WorkPlane4" through (0, 0, -7.475) normal (0, 0, 1) x (1, 0, 0) in component "04 Optical retainer"
sketch "Optical screw ear profile (1)" plane through (0, 0, -7.475) normal (0, 0, 1) x (1, 0, 0) in component "04 Optical retainer"
  line L0 (55.8, 47) -> (64.2, 47)
  line L1 (64.2, 47) -> (64.2, 57)
  line L2 (64.2, 57) -> (55.8, 57)
  line L3 (55.8, 57) -> (55.8, 47)
  dimension "d469" = 8.4
  dimension "d470" = 10
  measures "d469" horizontal distance of L0.start L0.end
  measures "d470" vertical distance of L0.end L1.end
extrude "Optical screw ear (1)" add sketch "Optical screw ear profile (1)" against normal blind 1.6 separate body makes body 55 in component "04 Optical retainer"
ref_plane "WorkPlane5" through (0, 0, -7.475) normal (0, 0, 1) x (1, 0, 0) in component "04 Optical retainer"